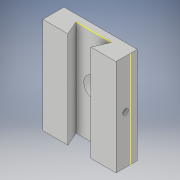
# Autodesk Inventor part: Schienenläuderaufsatz-22.11
Saved by Autodesk Inventor 2018.3 (Build 223284000, 284)
## iProperties
Created: 2018-10-11
Part Number: Schienenläuderaufsatz-22.11
Material: Generisch
Document SubType Name: Modeling
Designer: pgmadmin
Density: 1 g/cm^3
Appearance: Vorgabe
Author: pgmadmin
Autodesk Inventor part; units mm, degrees
ref_plane "YZ Plane" through (0, 0, 0) normal (1, 0, 0) x (0, 1, 0)
ref_plane "XZ Plane" through (0, 0, 0) normal (0, 1, 0) x (-1, 0, 0)
ref_plane "XY Plane" through (0, 0, 0) normal (0, 0, 1) x (1, 0, 0)
sketch "Skizze1" plane through (0, 0, 0) normal (0, 0, 1) x (1, 0, 0)
  line L0 (-18.1618, 0.375) -> (-21.3761, 7.875)
  line L1 (-2.9476, 7.875) -> (-6.1618, 0.375)
  line L2 (-6.1618, 0.375) -> (-18.1618, 0.375)
  line L3 (-18.1618, 0.375) -> (-31.1618, 0.375)
  line L4 (-31.1618, 0.375) -> (-31.1618, 11.375)
  line L5 (-31.1618, 11.375) -> (6.8382, 11.375)
  line L6 (6.8382, 11.375) -> (6.8382, 0.375)
  line L7 (6.8382, 0.375) -> (-6.1618, 0.375)
  line L8 (-21.5376, 7.875) -> (-2.9476, 7.875)
  point P0 (0, 0)
  point P1 (-21.1618, 7.375)
  point P2 (-3.1618, 7.375)
  dimension "d10" = 38
  dimension "d14" = 12
  dimension "d29" = 13
  constraints: 18 end point, 4 perpendicular, 4 point on line, 2 horizontal, 1 collinear
  measures "d10" distance of L4.end L5.end
  measures "d14" distance of L1.end L0.start
  measures "d29" distance of L0.start L3.end
extrude "Extrusion1" add sketch "Skizze1" along normal blind 50 contours L3 L4 L5 L6 L7 L1 L8 L0
sketch "Skizze2" plane through (6.8382, 0.375, 0) normal (1, 0, 0) x (0, 0, -1)
  line L0 (-50, 0) -> (-50, 11) projected
  line L1 (0, 11) -> (-50, 11) projected
  point P0 (0, -0.375)
  point P1 (-25, 4.85)
  dimension "d19" = 6.15
  measures "d19" distance from line of L1 point (-25, 4.85)
hole "Bohrung1" at (6.8382, 5.225, 25) direction (-1, 0, 0) diameter 2.9 depth 8 tip angle 118
sketch "Skizze3" plane through (-21.3761, 7.875, 0) normal (0, -1, 0) x (1, 0, 0)
  line L0 (0, 50) -> (18.4286, 50) projected
  line L1 (28.2143, 0) -> (28.2143, 50) projected
  point P0 (21.3761, 0)
sketch "Skizze4" plane through (-21.3761, 7.875, 0) normal (0, -1, 0) x (1, 0, 0)
  line L0 (0, 50) -> (18.4286, 50) projected
  line L1 (28.2143, 0) -> (28.2143, 50) projected
  point P0 (21.3761, 0)
  point P1 (9.2143, 25)
  dimension "d30" = 25
  dimension "d31" = 19
  measures "d30" distance from line of L0 point (9.214, 25)
  measures "d31" distance from line of L1 point (9.214, 25)
hole "Bohrung2" at (-12.1618, 7.875, 25) direction (0, 1, 0) diameter 5.2 end through all countersink diameter 10.5 countersink angle 90
